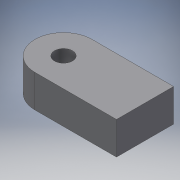
# Autodesk Inventor part: Motor Axle Fitting Test
Saved by Autodesk Inventor 2020 (Build 240168000, 168)
## iProperties
Created: 2020-02-06
Part Number: Motor Axle Fitting Test
Material: Generic
Document SubType Name: Modeling
Designer: Wes
Density: 1 g/cm^3
Appearance: Default
Author: Wes
Autodesk Inventor part; units mm, degrees
ref_plane "YZ Plane" through (0, 0, 0) normal (1, 0, 0) x (0, 1, 0)
ref_plane "XZ Plane" through (0, 0, 0) normal (0, 1, 0) x (-1, 0, 0)
ref_plane "XY Plane" through (0, 0, 0) normal (0, 0, 1) x (1, 0, 0)
sketch "Sketch1 - base" plane through (0, 0, 0) normal (0, 0, 1) x (1, 0, 0)
  circle A0 centre (0, 0) radius 3.5
  line L0 (-3.5, 0) -> (-3.5, 10)
  line L1 (-3.5, 10) -> (3.5, 10)
  line L2 (3.5, 10) -> (3.5, 0)
  dimension "d0" = 7
  dimension "d1" = 10
  constraints: 6 end point, 2 point on circle, 1 centre point, 1 horizontal, 1 perpendicular, 1 tangent, 1 vertical
  measures "d0" diameter of A0
  measures "d1" distance of L0.start L0.end
extrude "Extrusion1" add sketch "Sketch1 - base" along normal blind 4
sketch "Sketch2 - axle_hole" plane through (0, 0, 0) normal (0, 0, -1) x (-1, 0, 0)
  circle A0 centre (0, 0) radius 2.275
  line L0 (-2.247, 0.356) -> (-2.5426, 0.4069) construction
  arc A1 (-2.1625, 0.7067) -> (-2.275, 0) centre (-2.1883, 0.3485) ccw
  arc A2 (-2.275, 0.0038) -> (-2.1637, -0.703) centre (-2.1889, -0.3448) ccw
  arc A3 (-2.1648, -0.6994) -> (-1.8405, -1.3372) centre (-1.9752, -1.0043) ccw
  arc A4 (-1.8428, -1.3341) -> (-1.3372, -1.8405) centre (-1.5682, -1.5655) ccw
  arc A5 (-1.3403, -1.8382) -> (-0.703, -2.1637) centre (-1.0077, -1.9735) ccw
  arc A6 (-0.7067, -2.1625) -> (0, -2.275) centre (-0.3485, -2.1883) ccw
  arc A7 (-0.0038, -2.275) -> (0.703, -2.1637) centre (0.3448, -2.1889) ccw
  arc A8 (0.6994, -2.1648) -> (1.3372, -1.8405) centre (1.0043, -1.9752) ccw
  arc A9 (1.3341, -1.8428) -> (1.8405, -1.3372) centre (1.5655, -1.5682) ccw
  arc A10 (1.8382, -1.3403) -> (2.1637, -0.703) centre (1.9735, -1.0077) ccw
  arc A11 (2.1625, -0.7067) -> (2.275, 0) centre (2.1883, -0.3485) ccw
  arc A12 (2.275, -0.0038) -> (2.1637, 0.703) centre (2.1889, 0.3448) ccw
  arc A13 (2.1648, 0.6994) -> (1.8405, 1.3372) centre (1.9752, 1.0043) ccw
  arc A14 (1.8428, 1.3341) -> (1.3372, 1.8405) centre (1.5682, 1.5655) ccw
  arc A15 (1.3403, 1.8382) -> (0.703, 2.1637) centre (1.0077, 1.9735) ccw
  arc A16 (0.7067, 2.1625) -> (0, 2.275) centre (0.3485, 2.1883) ccw
  arc A17 (0.0038, 2.275) -> (-0.703, 2.1637) centre (-0.3448, 2.1889) ccw
  arc A18 (-0.6994, 2.1648) -> (-1.3372, 1.8405) centre (-1.0043, 1.9752) ccw
  arc A19 (-1.3341, 1.8428) -> (-1.8405, 1.3372) centre (-1.5655, 1.5682) ccw
  arc A20 (-1.8382, 1.3403) -> (-2.1637, 0.703) centre (-1.9735, 1.0077) ccw
  point P0 (-2.5439, -0.3988)
  point P1 (-2.2962, -1.1654)
  point P2 (-1.8237, -1.8179)
  point P3 (-1.1727, -2.2925)
  point P4 (-0.4069, -2.5426)
  point P5 (0.3988, -2.5439)
  point P6 (1.1654, -2.2962)
  point P7 (1.8179, -1.8237)
  point P8 (2.2925, -1.1727)
  point P9 (2.5426, -0.4069)
  point P10 (2.5439, 0.3988)
  point P11 (2.2962, 1.1654)
  point P12 (1.8237, 1.8179)
  point P13 (1.1727, 2.2925)
  point P14 (0.4069, 2.5426)
  point P15 (-0.3988, 2.5439)
  point P16 (-1.1654, 2.2962)
  point P17 (-1.8179, 1.8237)
  point P18 (-2.2925, 1.1727)
  point P19 (-2.2824, 0.0019)
  point P20 (-2.1713, -0.7035)
  point P21 (-1.8476, -1.34)
  point P22 (-1.3431, -1.8454)
  point P23 (-0.7071, -2.1701)
  point P24 (-0.0019, -2.2824)
  point P25 (0.7035, -2.1713)
  point P26 (1.34, -1.8476)
  point P27 (1.8454, -1.3431)
  point P28 (2.1701, -0.7071)
  point P29 (2.2824, -0.0019)
  point P30 (2.1713, 0.7035)
  point P31 (1.8476, 1.34)
  point P32 (1.3431, 1.8454)
  point P33 (0.7071, 2.1701)
  point P34 (0.0019, 2.2824)
  point P35 (-0.7035, 2.1713)
  point P36 (-1.34, 1.8476)
  point P37 (-1.8454, 1.3431)
  point P38 (-2.1701, 0.7071)
  dimension "d4" = 4.55
  dimension "d5" = 0.3
  dimension "d8" = 360
  constraints: 63 point on circle, 21 centre point, 2 end point, 1 coincident, 101 other
  measures "d4" diameter of A0
  measures "d5" distance of L0.start L0.end
extrude "Extrusion2" cut sketch "Sketch2 - axle_hole" against normal blind 2
sketch "Sketch3" plane through (0, 0, 0) normal (0, 0, -1) x (-1, 0, 0)
  circle A0 centre (0, 0) radius 1.1
  dimension "d12" = 2.2
  constraints: 1 centre point, 1 coincident
  measures "d12" diameter of A0
extrude "Extrusion3" cut sketch "Sketch3" against normal blind 4
body "Solid1"
